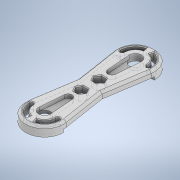
# Autodesk Inventor part: Upper_Limb
Saved by Autodesk Inventor 2021 (Build 250183000, 183)
## iProperties
Created: 2021-08-13
Part Number: Upper_Limb
Material: ABS Plastic
Document SubType Name: Modeling
Designer: rbnsmathew
Density: 1.06 g/cm^3
Appearance: Smooth - White
Mass: 6.3061 g
Surface Area: 48.7085 cm^2
Volume: 5.94915 cm^3
Author: rbnsmathew
Autodesk Inventor part; units mm, degrees
ref_plane "YZ Plane" through (0, 0, 0) normal (1, 0, 0) x (0, 1, 0)
ref_plane "XZ Plane" through (0, 0, 0) normal (0, 1, 0) x (-1, 0, 0)
ref_plane "XY Plane" through (0, 0, 0) normal (0, 0, 1) x (1, 0, 0)
sketch "Sketch2" plane through (0, 0, 0) normal (0, 1, 0) x (-1, 0, 0)
  line L0 (0, 0) -> (0, 30)
  line L1 (0, 0) -> (0, -30)
  circle A0 centre (0, 30) radius 3.9
  circle A1 centre (0, -30) radius 3.9
  circle A2 centre (0, 30) radius 9
  circle A3 centre (0, 30) radius 12.5
  circle A4 centre (0, -30) radius 9
  circle A5 centre (0, -30) radius 12.5
  line L2 (0, 0) -> (8, 0)
  line L3 (0, 0) -> (-8, 0)
  line L4 (8, 0) -> (12.3525, 28.0857)
  line L5 (8, 0) -> (12.3525, -28.0857)
  line L6 (-8, 0) -> (-12.3525, -28.0857)
  line L7 (-8, 0) -> (-12.3525, 28.0857)
  dimension "d0" = 30
  dimension "d1" = 30
  dimension "d2" = 7.8
  dimension "d3" = 7.8
  dimension "d4" = 18
  dimension "d5" = 25
  dimension "d6" = 25
  dimension "d7" = 18
  dimension "d8" = 8
  dimension "d9" = 8
  constraints: 16 end point, 6 centre point, 6 coincident, 4 point on circle, 4 tangent, 4 vertical, 2 horizontal
  measures "d0" distance of L0.start L0.end
  measures "d1" distance of L0.start L1.end
  measures "d2" diameter of A0
  measures "d3" diameter of A1
  measures "d4" diameter of A2
  measures "d5" diameter of A3
  measures "d6" diameter of A5
  measures "d7" diameter of A4
  measures "d8" distance of L0.start L2.end
  measures "d9" distance of L0.start L3.end
extrude "Extrusion1" add sketch "Sketch2" along normal blind 1.8 contours L3 L7 A3 L0 | L2 L5 A5 L1 | L0 A3 L4 L2 | L1 A5 L6 L3 | A3 | A5 | A2 | A4
sketch "Sketch3" plane through (0, 0, 0) normal (0, -1, 0) x (1, 0, 0)
  line L0 (12.3525, 28.0857) -> (8, 0) projected
  arc A0 (12.3525, 28.0857) -> (-12.3525, 28.0857) centre (0, 30) ccw projected
  line L1 (-8, 0) -> (-12.3525, 28.0857) projected
  line L2 (-12.3525, -28.0857) -> (-8, 0) projected
  arc A1 (-12.3525, -28.0857) -> (12.3525, -28.0857) centre (0, -30) ccw projected
  line L3 (8, 0) -> (12.3525, -28.0857) projected
  circle A2 centre (0, -30) radius 3.9 projected
  circle A3 centre (0, 30) radius 3.9 projected
  arc A4 (10, 30) -> (-10, 30) centre (0, 30) ccw
  arc A5 (-10, -30) -> (10, -30) centre (0, -30) ccw
  arc A6 (12.3525, 28.0857) -> (-12.3525, 28.0857) centre (0, 30) ccw projected
  circle A7 centre (0, 30) radius 3.9 projected
  arc A8 (-12.3525, -28.0857) -> (12.3525, -28.0857) centre (0, -30) ccw projected
  line L4 (-3.3508, 30) -> (-3.9, 30)
  line L5 (-10, 30) -> (-12.5, 30)
  line L6 (3.3508, 30) -> (3.9, 30)
  line L7 (10, 30) -> (12.5, 30)
  line L8 (3.3508, -30) -> (3.9, -30)
  line L9 (10, -30) -> (12.5, -30)
  line L10 (-3.3508, -30) -> (-3.9, -30)
  line L11 (-10, -30) -> (-12.5, -30)
  point P0 (0, 0)
  dimension "d12" = 20
  dimension "d13" = 20
  constraints: 16 end point, 12 point on circle, 4 parallel, 4 point on line, 2 centre point, 2 coincident, 2 horizontal
  measures "d12" diameter of A4
  measures "d13" diameter of A5
extrude "Extrusion2" add sketch "Sketch3" along normal blind 2 contours L7 A4 L5 A0 | A1 L11 A5 L9
sketch "Sketch4" plane through (0, 1.8, 0) normal (0, 1, 0) x (1, 0, 0)
  line L0 (12.3525, -28.0857) -> (8, 0) projected
  line L1 (8, 0) -> (12.3525, 28.0857) projected
  arc A0 (12.3525, 28.0857) -> (-12.3525, 28.0857) centre (0, 30) ccw projected
  line L2 (-12.3525, 28.0857) -> (-8, 0) projected
  line L3 (-8, 0) -> (-12.3525, -28.0857) projected
  arc A1 (-12.3525, -28.0857) -> (12.3525, -28.0857) centre (0, -30) ccw projected
  circle A2 centre (0, 30) radius 3.9 projected
  circle A3 centre (0, -30) radius 3.9 projected
  circle A4 centre (0, 30) radius 3.9 projected
  line L4 (0, 30) -> (0, 14.5)
  line L5 (0, -30) -> (0, -14.5)
  arc A5 (-2.6414, 14.2863) -> (2.6414, 14.2863) centre (0, 14.5) ccw
  arc A6 (2.6414, -14.2863) -> (-2.6414, -14.2863) centre (0, -14.5) ccw
  line L6 (3.8873, 29.6855) -> (2.6414, 14.2863)
  line L7 (-2.6414, 14.2863) -> (-3.8873, 29.6855)
  line L8 (-2.6414, -14.2863) -> (-3.8873, -29.6855)
  line L9 (2.6414, -14.2863) -> (3.8873, -29.6855)
  circle A7 centre (0, -30) radius 3.9 projected
  point P0 (0, 0)
  point P1 (-3.8873, 29.6855)
  point P2 (3.8873, 29.6855)
  point P3 (-3.8873, -29.6855)
  dimension "d16" = 15.5
  dimension "d17" = 15.5
  dimension "d18" = 5.3
  dimension "d19" = 5.3
  constraints: 12 end point, 8 point on circle, 8 tangent, 2 centre point, 2 coincident, 2 vertical
  measures "d16" distance of L4.start L4.end
  measures "d17" distance of L5.start L5.end
  measures "d18" diameter of A5
  measures "d19" diameter of A6
extrude "Extrusion3" add sketch "Sketch4" along normal blind 2.5
sketch "Sketch5" plane through (0, 0, 0) normal (0, -1, 0) x (1, 0, 0)
  line L0 (10, -30) -> (12.5, -30) projected
  arc A0 (12.5, -30) -> (12.3525, -28.0857) centre (0, -30) ccw projected
  line L1 (8, 0) -> (12.3525, -28.0857) projected
  line L2 (12.3525, 28.0857) -> (8, 0) projected
  arc A1 (12.3525, 28.0857) -> (12.5, 30) centre (0, 30) ccw projected
  line L3 (12.5, 30) -> (10, 30) projected
  arc A2 (10, 30) -> (-10, 30) centre (0, 30) ccw projected
  line L4 (-10, 30) -> (-12.5, 30) projected
  arc A3 (-12.5, 30) -> (-12.3525, 28.0857) centre (0, 30) ccw projected
  line L5 (-8, 0) -> (-12.3525, 28.0857) projected
  line L6 (-12.3525, -28.0857) -> (-8, 0) projected
  arc A4 (-12.3525, -28.0857) -> (-12.5, -30) centre (0, -30) ccw projected
  line L7 (-12.5, -30) -> (-10, -30) projected
  arc A5 (-10, -30) -> (10, -30) centre (0, -30) ccw projected
  circle A6 centre (0, -30) radius 3.9 projected
  circle A7 centre (0, 30) radius 3.9 projected
  circle A8 centre (0, -30) radius 10
  arc A9 (-7.5, -30) -> (7.5, -30) centre (0, -30) ccw
  line L8 (0, -30) -> (-10, -30)
  line L9 (10, -30) -> (0, -30)
  line L10 (0, -30) -> (-2.5882, -39.6593)
  arc A10 (-10, -30) -> (10, -30) centre (0, -30) ccw projected
  line L11 (0, -30) -> (2.5882, -39.6593)
  line L12 (0, -30) -> (0, -40)
  circle A11 centre (0, 30) radius 3.9 projected
  circle A12 centre (0, 30) radius 10
  arc A13 (7.5, 30) -> (-7.5, 30) centre (0, 30) ccw
  line L13 (-10, 30) -> (-12.5, 30) projected
  line L14 (0, 30) -> (-10, 30)
  line L15 (-10, 30) -> (0, 30)
  line L16 (10, 30) -> (0, 30)
  line L17 (0, 30) -> (0, 40)
  arc A14 (10, 30) -> (-10, 30) centre (0, 30) ccw projected
  line L18 (0, 30) -> (-2.5882, 39.6593)
  line L19 (0, 30) -> (2.5882, 39.6593)
  line L20 (-7.5, -30) -> (-10, -30)
  circle A15 centre (8.75, -30) radius 1.25
  circle A16 centre (-8.75, -30) radius 1.25
  circle A17 centre (-8.75, 30) radius 1.25
  circle A18 centre (8.75, 30) radius 1.25
  point P0 (0, 0)
  point P1 (1.9411, 37.2444)
  point P2 (-1.9411, 37.2444)
  point P3 (1.9411, -37.2444)
  point P4 (-1.9411, -37.2444)
  dimension "d22" = 20
  dimension "d23" = 15
  dimension "d24" = 15
  dimension "d25" = 15
  dimension "d26" = 20
  dimension "d27" = 15
  dimension "d28" = 15
  dimension "d29" = 15
  dimension "d43" = 1.25
  dimension "d44" = 2.5
  dimension "d45" = 1.25
  dimension "d46" = 2.5
  dimension "d47" = 1.25
  dimension "d48" = 2.5
  dimension "d49" = 2.5
  dimension "d50" = 1.25
  constraints: 24 end point, 12 point on circle, 8 centre point, 7 point on line, 4 coincident, 4 collinear, 2 horizontal, 1 midpoint
  measures "d22" diameter of A8
  measures "d23" diameter of A9
  measures "d24" angle of L10 L12
  measures "d25" angle of L11 L12
  measures "d26" diameter of A12
  measures "d27" diameter of A13
  measures "d28" angle of L18 L17
  measures "d29" angle of L19 L17
  measures "d43" distance of A15.centre A9.end
  measures "d44" diameter of A15
  measures "d45" distance of L20.start A16.centre
  measures "d46" diameter of A16
  measures "d47" distance of A17.centre A13.end
  measures "d48" diameter of A17
  measures "d49" diameter of A18
  measures "d50" distance of A13.start A18.centre
extrude "Extrusion4" cut sketch "Sketch5" against normal blind 5 contours A15 L9 | L9 A15 | A5 L11 A9 A15 | A16 A9 L10 A5 | A16 L8 | L8 A16 | A18 A13 L19 A2 | A18 L16 | L16 A18 | A17 L14 | A2 L18 A13 A17 | L14 A17
sketch "Sketch6" plane through (0, 4.3, 0) normal (0, 1, 0) x (1, 0, 0)
  line L0 (0, 0) -> (0, 6)
  line L1 (0, 6) -> (0, 0)
  line L2 (0, 0) -> (0, -6)
  circle A0 centre (0, -6) radius 3.5
  circle A1 centre (0, 6) radius 3.5
  line L3 (-3.5, -6) -> (-1.75, -2.9689)
  line L4 (-1.75, -2.9689) -> (1.75, -2.9689)
  line L5 (1.75, -2.9689) -> (3.5, -6)
  line L6 (3.5, -6) -> (1.75, -9.0311)
  line L7 (1.75, -9.0311) -> (-1.75, -9.0311)
  line L8 (-1.75, -9.0311) -> (-3.5, -6)
  line L9 (-3.4979, 6.1207) -> (-1.6444, 9.0897)
  line L10 (-1.6444, 9.0897) -> (1.8535, 8.9689)
  line L11 (1.8535, 8.9689) -> (3.4979, 5.8793)
  line L12 (3.4979, 5.8793) -> (1.6444, 2.9103)
  line L13 (1.6444, 2.9103) -> (-1.8535, 3.0311)
  line L14 (-1.8535, 3.0311) -> (-3.4979, 6.1207)
  dimension "d34" = 7
  dimension "d35" = 7
  dimension "d32" = 6
  dimension "d33" = 6
  constraints: 30 end point, 4 coincident, 2 point on line, 1 collinear, 1 horizontal alignment, 1 vertical, 31 other
  measures "d32" distance of L0.start L2.end
  measures "d33" distance of L0.start L0.end
extrude "Extrusion5" cut sketch "Sketch6" against normal blind 5 contours L13 L14 L9 L10 L11 L12 | L4 L5 L6 L7 L8 L3
chamfer "Chamfer1" distance 1.5 angle 45 6 edges at (10.1763, 4.3, -14.0428) (0, 4.3, -42.5) (-10.1763, 4.3, -14.0428) (10.1763, 4.3, 14.0428) (0, 4.3, 42.5) (-10.1763, 4.3, 14.0428)
chamfer "Chamfer2" distance 0.5 angle 45 28 edges at (-5.9502, 4.3, 34.5657) (-8.75, 4.3, 28.75) (-7.9335, 4.3, 36.0876) (-2.2647, 4.3, 38.4519) (2.2647, 4.3, 38.4519) (7.9335, 4.3, 36.0876) (8.75, 4.3, 28.75) (5.9502, 4.3, 34.5657) (-5.9502, 4.3, -34.5657) (-8.75, 4.3, -28.75) (-7.9335, 4.3, -36.0876) (-2.2647, 4.3, -38.4519) (2.2647, 4.3, -38.4519) (5.9502, 4.3, -34.5657) (8.75, 4.3, -28.75) (7.9335, 4.3, -36.0876) (0, 4.3, 9.0311) (-2.625, 4.3, 7.5155) (-2.625, 4.3, 4.4845) (0, 4.3, 2.9689) (2.625, 4.3, 4.4845) (2.625, 4.3, 7.5155) (-0.1046, 4.3, -2.9707) (-2.6757, 4.3, -4.5759) (-2.5712, 4.3, -7.6052) (0.1046, 4.3, -9.0293) (2.6757, 4.3, -7.4241) (2.5712, 4.3, -4.3948)
equation "\"d1\" = d0"
equation "\"d6\" = d5"
equation "\"d7\" = d4"
equation "\"d9\" = d8"
equation "\"d17\" = d16"
equation "\"d19\" = d18"
body "Solid1"
